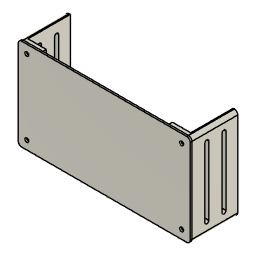
V3.1_Radio Stack PCB System v9 (Autodesk Fusion 360 design; units mm, degrees)
Autodesk Fusion 360 part; units mm, degrees
note: some values were not read from the file. Set by a fixed rule: which sketch regions a step uses.
sketch "Sketch1" plane through (0, 0, 0) normal (0, 1, 0) x (1, 0, 0) in component "PCB Profile"
  line L0 (72, -40) -> (-72, -40)
  line L1 (-75, -37) -> (-75, 37)
  line L2 (-72, 40) -> (72, 40)
  line L3 (75, 37) -> (75, -37)
  line L4 (75, -40) -> (-75, 40) construction
  line L5 (-75, -40) -> (75, 40) construction
  arc A0 (-75, -37) -> (-72, -40) centre (-72, -37) ccw
  arc A1 (72, -40) -> (75, -37) centre (72, -37) ccw
  arc A2 (75, 37) -> (72, 40) centre (72, 37) ccw
  arc A3 (-72, 40) -> (-75, 37) centre (-72, 37) ccw
  circle A4 centre (67.5, -32.5) radius 1.75
  line L6 (0, 0) -> (0, -40) construction
  line L7 (0, 0) -> (-75, 0) construction
  circle A5 centre (-67.5, -32.5) radius 1.75
  circle A6 centre (-67.5, 32.5) radius 1.75
  circle A7 centre (67.5, 32.5) radius 1.75
  point P0 (-67.5, -32.5)
  dimension "d1" = 3
  dimension "d2" = 150
  dimension "d3" = 80
  dimension "d8" = 3.5
  dimension "d9" = 67.5
  dimension "d10" = 32.5
  dimension "d16" = 7.5
  dimension "d17" = 7.5
  constraint horizontal L0
  constraint perpendicular L0 L1
  constraint parallel L0 L2
  constraint parallel L1 L3
  constraint coincident L4 L6.start
  constraint coincident L5 L6.start
  constraint coincident L6.start L7.start
  constraint coincident L5.start L1
  constraint coincident L5.start L0
  constraint tangent L1 A0
  constraint tangent L0 A0
  constraint coincident L4.start L0
  constraint coincident L4.start L3
  constraint tangent L0 A1
  constraint tangent L3 A1
  constraint equal A0 A1
  constraint coincident L5.end L2
  constraint coincident L5.end L3
  constraint tangent L2 A2
  constraint tangent L3 A2
  constraint equal A0 A2
  constraint coincident L4.end L2
  constraint coincident L4.end L1
  constraint tangent L2 A3
  constraint tangent L1 A3
  constraint equal A0 A3
  constraint midpoint L0 L6.end
  constraint symmetric A4.centre L6 P0
  constraint midpoint L1 L7.end
  constraint symmetric A4 L6 A5
  constraint symmetric A4 L7 A7
  constraint symmetric L7 A5 A6
  measures "d1" radius of A0
  measures "d2" distance of L1 L3
  measures "d3" distance of L0 L2
  measures "d8" diameter of A4
  measures "d9" horizontal distance of L6.start A4.centre
  measures "d10" vertical distance of L6.start A4.centre
  measures "d16" distance of L0 A4.centre
  measures "d17" distance of L3 A4.centre
extrude "Extrude1" add sketch "Sketch1" along normal blind 1.5 makes body 1 in component "PCB Profile"
sketch "Sketch1 (2)" plane through (0, 1.5, 0) normal (0, 1, 0) x (-1, 0, 0) in component "Rack Mounts"
  arc A0 (-75, -37) -> (-72, -40) centre (-72, -37) ccw
  line L0 (-72, -40) -> (72, -40)
  arc A1 (72, -40) -> (75, -37) centre (72, -37) ccw
  line L1 (75, -37) -> (75, 37)
  arc A2 (75, 37) -> (72, 40) centre (72, 37) ccw
  line L2 (72, 40) -> (-72, 40)
  arc A3 (-72, 40) -> (-75, 37) centre (-72, 37) ccw
  line L3 (-75, 37) -> (-75, -37)
  line L4 (-55, 40) -> (-55, -40)
  line L5 (55, 40) -> (55, -40)
  circle A4 centre (-67.5, 32.5) radius 1.75
  circle A5 centre (-67.5, -32.5) radius 1.75
  circle A6 centre (67.5, -32.5) radius 1.75
  circle A7 centre (67.5, 32.5) radius 1.75
  line L6 (-71, 40) -> (-71, -40)
  dimension "d6" = 20
  dimension "d7" = 20
  dimension "d11" = 4
  constraint coincident L2 L4.start
  constraint perpendicular L2 L4
  constraint coincident L2 L5.start
  constraint coincident L0 L5.end
  constraint perpendicular L0 L5
  constraint coincident L0 L4.end
  constraint coincident L2 L6.start
  constraint coincident L0 L6.end
  constraint perpendicular L0 L6
  measures "d6" distance of L1 L5
  measures "d7" distance of L3 L4
  measures "d11" distance of L3 L6
extrude "Extrude1'" add sketch "Sketch1 (2)" along normal blind 40 separate body contours A0 L0 L2 A3 L3 L6 makes body 2 in component "Rack Mounts"
extrude "Extrude2" add sketch "Sketch1 (2)" along normal blind 3 contours L0 L2 L4 L6 bodies 2 in component "Rack Mounts"
mirror "Mirror1" about plane through (0, 0, 0) normal (1, 0, 0) of bodies 2 makes body 3 in component "Rack Mounts"
sketch "Sketch2" plane through (-75, 0, 0) normal (-1, 0, 0) x (0, -1, 0) in component "Rack Mounts"
  line L0 (-1.5, -37) -> (-1.5, 37)
  line L1 (-1.5, 37) -> (-41.5, 37)
  line L2 (-41.5, 37) -> (-41.5, -37)
  line L3 (-41.5, -37) -> (-1.5, -37)
  line L4 (-31.25, 30) -> (-31.25, -30)
  arc A0 (-31.25, -30) -> (-27.75, -30) centre (-29.5, -30) ccw
  line L5 (-27.75, -30) -> (-27.75, 30)
  arc A1 (-27.75, 30) -> (-31.25, 30) centre (-29.5, 30) ccw
  line L6 (-29.5, 30) -> (-29.5, -30) construction
  line L7 (-16.25, 30) -> (-16.25, -30)
  arc A2 (-16.25, -30) -> (-12.75, -30) centre (-14.5, -30) ccw
  line L8 (-12.75, -30) -> (-12.75, 30)
  arc A3 (-12.75, 30) -> (-16.25, 30) centre (-14.5, 30) ccw
  line L9 (-14.5, 30) -> (-14.5, -30) construction
  line L10 (-1.5, -40) -> (-41.5, -40)
  line L11 (-1.5, 40) -> (-41.5, 40)
  point P0 (-4.5, 40)
  dimension "d20" = 1.75
  dimension "d21" = 15
  dimension "d22" = 10
  dimension "d23" = 10
  dimension "d24" = 10
  constraint tangent L4 A0
  constraint tangent A0 L5
  constraint parallel L4 L5
  constraint tangent L5 A1
  constraint tangent L4 A1
  constraint vertical L6
  constraint tangent L7 A2
  constraint tangent A2 L8
  constraint parallel L7 L8
  constraint tangent L8 A3
  constraint tangent L7 A3
  constraint parallel L5 L9
  constraint equal A0 A2
  constraint horizontal A0.centre A2.centre
  constraint horizontal A1.centre A3.centre
  measures "d20" radius of A0
  measures "d21" distance of L6 L9
  measures "d22" distance of A0.centre L10
  measures "d23" distance of A1.centre L11
  measures "d24" horizontal distance of A3.centre P0
extrude "Extrude3" cut sketch "Sketch2" against normal through all contours L4 A0 L5 A1 | L7 A2 L8 A3 bodies 2 3 in component "Rack Mounts"
component "PCB Profile" placed x (1, 0, 0) y (0, 1, 0) z (0, 0, 1) at (0, 0, 0)
component "Rack Mounts" placed x (1, 0, 0) y (0, 1, 0) z (0, 0, 1) at (0, 0, 0)
equation "d7 = d6"
equation "d20 = ( 3.5 / 2 ) * 1 mm"
named bodies: "Rack Mount x2"
